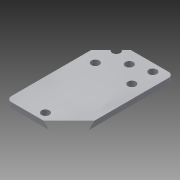
# Autodesk Inventor part: Roller Pneumatic Back Connector (Custom)
Saved by Autodesk Inventor 2014 (Build 180170000, 170)
## iProperties
Created: 2014-01-06
Part Number: Roller Pneumatic Back Connector (Custom)
Material: Aluminum 6061
Document SubType Name: Modeling
Designer: Andrew Toennies
Density: 7.85 g/cm^3
Appearance: Aluminum - Flat
Mass: 11.2814 g
Surface Area: 21.4027 cm^2
Volume: 1.43712 cm^3
Author: Andrew Toennies
Autodesk Inventor part; units mm, degrees
ref_plane "YZ Plane" through (0, 0, 0) normal (1, 0, 0) x (0, 1, 0)
ref_plane "XZ Plane" through (0, 0, 0) normal (0, 1, 0) x (-1, 0, 0)
ref_plane "XY Plane" through (0, 0, 0) normal (0, 0, 1) x (1, 0, 0)
sketch "Sketch1" plane through (0, 0, 0) normal (0, 1, 0) x (-1, 0, 0)
  circle A0 centre (0, 0) radius 2.413
  circle A1 centre (0, 50.8) radius 2.413
  line L0 (0, 50.8) -> (0, 0) construction
  circle A2 centre (11.049, 9.525) radius 2.413
  circle A3 centre (11.049, -3.175) radius 2.413
  circle A4 centre (-11.049, -3.175) radius 2.413
  circle A5 centre (-11.049, 9.525) radius 2.413
  line L1 (-11.049, -3.175) -> (-11.049, 9.525) construction
  line L2 (-11.049, 9.525) -> (11.049, 9.525) construction
  line L3 (-19.05, -7.9375) -> (19.05, -7.9375)
  line L4 (19.05, -7.9375) -> (19.05, 55.5625)
  line L5 (19.05, 55.5625) -> (-19.05, 55.5625)
  line L6 (-19.05, 55.5625) -> (-19.05, -7.9375)
  point P0 (0, 25.4)
  dimension "d1" = 4.826
  dimension "d2" = 50.8
  dimension "d3" = 4.826
  dimension "d4" = 4.826
  dimension "d5" = 12.7
  dimension "d6" = 11.049
  dimension "d7" = 11.049
  dimension "d9" = 4.826
  dimension "d10" = 4.826
  dimension "d11" = 11.049
  dimension "d12" = 12.7
  dimension "d18" = 7.9375
  dimension "d20" = 38.1
  dimension "d21" = 63.5
  dimension "d23" = 3.175
  constraints: 14 end point, 6 centre point, 3 parallel, 2 perpendicular, 1 coincident, 1 equal radius, 1 midpoint, 1 vertical, 1 other
  measures "d1" diameter of A1
  measures "d2" distance of L0.start L0.end
  measures "d3" diameter of A2
  measures "d4" diameter of A3
  measures "d5" distance of A3.centre L2.end
  measures "d6" distance from line of L0 A3.centre
  measures "d7" distance from line of L0 L2.end
  measures "d9" diameter of A4
  measures "d10" diameter of A5
  measures "d11" distance between parallel lines of L1 L0
  measures "d12" distance of L1.start L1.end
  measures "d18" distance from line of L3 point (0, 0)
  measures "d20" distance of L3.start L3.end
  measures "d21" distance of L5.end L3.start
  measures "d23" vertical distance of A3.centre L0.end
extrude "Extrusion1" add sketch "Sketch1" along normal blind 3.175
fillet "Fillet1" radius 3.175 4 edges at (19.05, 1.5875, 55.5625) (-19.05, 1.5875, 55.5625) (19.05, 1.5875, -7.9375) (-19.05, 1.5875, -7.9375)
equation "\"d7\" = d6"
equation "\"d11\" = d6"
body "Solid1"
